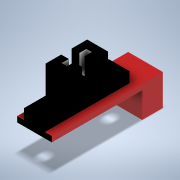
# Autodesk Inventor part: photointerrupter
Saved by Autodesk Inventor 2020 (Build 240168000, 168)
## iProperties
Created: 2020-02-12
Part Number: photointerrupter
Material: Generic
Document SubType Name: Modeling
Designer: LENOVO
Density: 1 g/cm^3
Appearance: Default
Author: LENOVO
Autodesk Inventor part; units mm, degrees
ref_plane "YZ Plane" through (0, 0, 0) normal (1, 0, 0) x (0, 1, 0)
ref_plane "XZ Plane" through (0, 0, 0) normal (0, 1, 0) x (-1, 0, 0)
ref_plane "XY Plane" through (0, 0, 0) normal (0, 0, 1) x (1, 0, 0)
sketch "Sketch1" plane through (0, 0, 0) normal (0, 1, 0) x (-1, 0, 0)
  circle A0 centre (0, 9.5) radius 1.5
  circle A1 centre (0, -9.5) radius 1.5
  line L0 (-3, 6) -> (3, 6)
  line L1 (3, 6) -> (3, -6)
  line L2 (3, -6) -> (-3, -6)
  line L3 (-3, -6) -> (-3, 6)
  line L4 (-3, 6) -> (3, -6) construction
  line L5 (3, 6) -> (-3, -6) construction
  line L6 (3, 12.2) -> (-3, 12.2)
  line L7 (-3, 12.2) -> (-3, -12.2)
  line L8 (-3, -12.2) -> (3, -12.2)
  line L9 (3, -12.2) -> (3, 12.2)
  line L10 (3, 12.2) -> (-3, -12.2) construction
  line L11 (-3, 12.2) -> (3, -12.2) construction
  line L12 (0, 12.2) -> (5, 12.2)
  line L13 (0, 12.2) -> (-5, 12.2)
  line L14 (-5, 12.2) -> (-5, -19.8)
  line L15 (-5, -19.8) -> (5, -19.8)
  line L16 (5, -19.8) -> (5, 12.2)
  line L17 (5, -19.8) -> (-0.01, -19.8)
  line L18 (4.99, -13.83) -> (-5.01, -13.83)
  line L19 (-5.01, -13.83) -> (-5.01, -19.83)
  line L20 (-5.01, -19.83) -> (4.99, -19.83)
  line L21 (4.99, -19.83) -> (4.99, -13.83)
  line L22 (4.99, -13.83) -> (-5.01, -19.83) construction
  line L23 (-5.01, -13.83) -> (4.99, -19.83) construction
  line L24 (3, 6) -> (3, 1.5)
  line L25 (3, 1.5) -> (-3, 1.5)
  line L26 (-3, 6) -> (3, 6)
  line L27 (-3, 6) -> (-3, 1.5)
  line L28 (3, -6) -> (3, -1.5)
  line L29 (3, -1.5) -> (-3, -1.5)
  line L30 (-3, -1.5) -> (-3, -6)
  line L31 (-3, -6) -> (3, -6)
  line L32 (-0.01, -16.83) -> (-0.01, -19.8)
  point P0 (0, 0)
  point P1 (0, 0)
  point P2 (0, -30.9776)
  point P3 (-5, -13.83)
  point P4 (-5, -19.33)
  point P5 (4.99, -19.8)
  dimension "d0" = 3
  dimension "d1" = 3
  dimension "d2" = 19
  dimension "d3" = 6
  dimension "d4" = 12
  dimension "d5" = 3.5
  dimension "d6" = 3.5
  dimension "d7" = 6
  dimension "d8" = 24.4
  dimension "d11" = 5
  dimension "d12" = 5
  dimension "d13" = 32
  dimension "d14" = 90
  dimension "d15" = 10
  dimension "d16" = 5.01
  dimension "d18" = 10
  dimension "d19" = 6
  dimension "d20" = 4.5
  dimension "d21" = 4.5
  constraints: 66 end point, 7 parallel, 7 perpendicular, 6 midpoint, 6 point on line, 4 horizontal, 2 centre point, 1 vertical
  measures "d0" diameter of A0
  measures "d1" diameter of A1
  measures "d2" distance of A0.centre A1.centre
  measures "d3" distance of L2.start L2.end
  measures "d4" distance of L1.start L2.start
  measures "d5" distance from line of A0.centre L0
  measures "d6" distance from line of L2 A1.centre
  measures "d7" distance of L8.end L7.end
  measures "d8" distance of L7.end L6.end
  measures "d11" distance of L12.start L12.end
  measures "d12" distance of L12.start L13.end
  measures "d13" distance of L13.end L14.end
  measures "d14" angle of L14 L13
  measures "d15" distance of L14.end L15.end
  measures "d16" distance of L15.end L17.end
  measures "d18" distance of L20.end L19.end
  measures "d19" distance of L19.end L18.end
  measures "d20" distance of L1.start L24.end
  measures "d21" distance of L2.start L28.end
extrude "Extrusion5" add sketch "Sketch1" against normal blind 1.6 contours A0 | A1 | L7 L6 L9 L0 | L0 L1 L25 L3 | L3 L7 L8 L9 L1 L12 L16 L15 L21 L18 L14 L13 | L25 L1 L29 L3 | L29 L1 L2 L3 | L2 L9 L8 L7 | L18 L21 L15 L14
extrude "Extrusion6" cut sketch "Sketch1" along normal mid plane 10 contours A0
extrude "Extrusion7" cut sketch "Sketch1" along normal mid plane 10 contours A1
extrude "Extrusion8" add sketch "Sketch1" along normal blind 3 contours L7 L6 L9 L0
extrude "Extrusion9" add sketch "Sketch1" along normal blind 3 contours L2 L9 L8 L7
extrude "Extrusion10" add sketch "Sketch1" against normal blind 9 contours L18 L21 L15 L14
extrude "Extrusion11" add sketch "Sketch1" along normal blind 3 contours L25 L1 L29 L3
extrude "Extrusion12" add sketch "Sketch1" along normal blind 11 contours L0 L1 L25 L3
extrude "Extrusion13" add sketch "Sketch1" along normal blind 11 contours L29 L1 L2 L3
sketch "Sketch2" plane through (-3, 3, -1.5) normal (0, 0, 1) x (1, 0, 0)
  line L0 (0, 8) -> (6, 8) projected
  line L1 (0, 8) -> (2.25, 8)
  line L2 (0, -3) -> (6, -3) projected
  line L3 (2.25, 8) -> (2.25, 3)
  line L4 (2.25, 3) -> (3.75, 3)
  line L5 (3.75, 3) -> (3.75, 8)
  line L6 (3.75, 8) -> (6, 8)
  line L7 (2.25, 8) -> (3.75, 8)
  point P0 (3, -3)
  dimension "d48" = 2.25
  dimension "d49" = 5
  dimension "d50" = 1.5
  constraints: 12 end point, 3 perpendicular, 2 point on line, 1 collinear, 1 parallel
  measures "d48" distance of L0.start L1.end
  measures "d49" distance of L1.end L3.end
  measures "d50" distance of L3.end L4.end
extrude "Extrusion14" cut sketch "Sketch2" against normal blind 2
sketch "Sketch3" plane through (3, 3, 1.5) normal (0, 0, -1) x (-1, 0, 0)
  line L0 (0, 8) -> (6, 8) projected
  line L1 (0, 8) -> (2.25, 8)
  line L2 (2.25, 8) -> (2.25, 3)
  line L3 (3.75, 3) -> (3.75, 8) projected
  line L4 (2.25, 3) -> (3.75, 3)
  line L5 (3.75, 3) -> (3.75, 8)
  line L6 (3.75, 8) -> (2.25, 8)
  point P0 (3, -3)
  dimension "d53" = 2.25
  dimension "d54" = 5
  dimension "d55" = 1.5
  constraints: 10 end point, 2 perpendicular, 2 point on line
  measures "d53" distance of L0.start L1.end
  measures "d54" distance of L1.end L2.end
  measures "d55" distance of L2.end L3.start
extrude "Extrusion15" cut sketch "Sketch3" against normal blind 2
body "Solid2"
